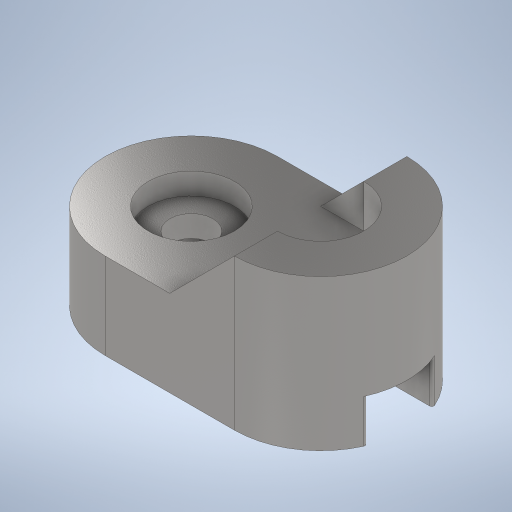
# Autodesk Inventor part: angel
Saved by Autodesk Inventor 2024 (Build 280153000, 153)
## iProperties
Created: 2024-02-01
Part Number: angel
Material: Stahl, galvanisiert
Document SubType Name: Modeling
Designer: ffogue
Density: 7.85 g/cm^3
Appearance: Galvanisiert
Author: ffogue
Autodesk Inventor part; units mm, degrees
note: some values were not read from the file. Chosen so that the rebuilt part matches the saved one: direction of "Bohrung1"; direction of "Bohrung2".
ref_plane "XY Plane" through (0, 0, 0) normal (0, 0, 1) x (1, 0, 0)
sketch "Skizze1" plane through (0, 0, 0) normal (0, 0, 1) x (1, 0, 0)
  line L0 (-70, 0) -> (70, 0) construction
  line L1 (-70, 40) -> (70, 40)
  line L2 (-70, -40) -> (70, -40)
  line L3 (-70, 40) -> (-70, -40)
  line L4 (70, 40) -> (70, -40)
  line L5 (0, 0) -> (0, 9.5703) construction
  dimension "d0" = 80
  dimension "d1" = 140
  constraints: 12 end point, 4 parallel, 2 vertical, 1 coincident, 1 horizontal, 1 midpoint, 1 vertical alignment, 2 other
  measures "d0" distance between parallel lines of L2 L1
  measures "d1" distance of L1.start L1.end
extrude "Extrusion1" add sketch "Skizze1" along normal blind 40
fillet "Rundung1" radius 40 1 edges at (-70, 40, 20)
fillet "Rundung2" radius 40 1 edges at (-70, -40, 20)
fillet "Rundung3" radius 40 1 edges at (70, 40, 20)
fillet "Rundung4" radius 40 1 edges at (70, -40, 20)
sketch "Skizze4" plane through (0, 0, 40) normal (0, 0, 1) x (1, 0, 0)
  circle A0 centre (-30, 0) radius 20
  circle A1 centre (30, 0) radius 20
  line L0 (0, 0) -> (0, 40) construction
  arc A2 (30, -40) -> (30, 40) centre (30, 0) ccw projected
  line L1 (30, 40) -> (-30, 40) projected
  point P0 (70, 0)
  dimension "d10" = 40
  dimension "d11" = 40
  dimension "d12" = 60
  constraints: 2 centre point, 2 end point, 2 horizontal alignment, 1 midpoint, 1 point on circle, 1 symmetric about line, 1 vertical
  measures "d10" diameter of A0
  measures "d11" diameter of A1
  measures "d12" distance of A1.centre A0.centre
extrude "Extrusion2" cut sketch "Skizze4" against normal blind 10
sketch "Skizze5" plane through (-30, 0, 30) normal (0, 0, 1) x (1, 0, 0)
  circle A0 centre (0, 0) radius 20 projected
  point P0 (30, 0)
  constraints: 1 coincident
hole "Bohrung1" at (-30, 0, 30) direction (0, 0, -1) diameter 20 depth 30
sketch "Skizze6" plane through (30, 0, 30) normal (0, 0, 1) x (1, 0, 0)
  circle A0 centre (0, 0) radius 20 projected
  point P0 (-30, 0)
  constraints: 1 coincident
hole "Bohrung2" at (30, 0, 30) direction (0, 0, -1) diameter 20 depth 30
sketch "Skizze7" plane through (0, 0, 40) normal (0, 0, 1) x (1, 0, 0)
  circle A0 centre (30, 0) radius 10 projected
  arc A1 (30, -40) -> (30, 40) centre (30, 0) ccw projected
  line L0 (30, 40) -> (-30, 40) projected
  arc A2 (30, -40) -> (30, 40) centre (30, 0) ccw
  circle A3 centre (30, 0) radius 20 projected
  arc A4 (30, -20) -> (30, 20) centre (30, 0) ccw
  line L1 (30, 40) -> (30, 20)
  line L2 (30, -20) -> (30, -40)
  point P0 (0, 0)
  constraints: 6 point on circle, 4 end point, 2 centre point, 2 vertical
extrude "Extrusion3" add sketch "Skizze7" along normal blind 30 contours L2 A3 L1 A1
sketch "Skizze8" plane through (-30, -40, 0) normal (0, -1, 0) x (1, 0, 0)
  line L0 (60, 40) -> (60, 70) projected
  line L1 (0, 40) -> (60, 40) projected
  line L2 (60, 70) -> (30, 40)
  line L3 (60, 40) -> (30, 40)
  line L4 (60, 40) -> (60, 70) projected
  line L5 (60, 70) -> (60, 40)
  point P0 (30, 0)
  dimension "d31" = 30
  constraints: 6 end point, 2 collinear, 1 midpoint
  measures "d31" distance of L0.start L2.end
extrude "Extrusion4" add sketch "Skizze8" against normal blind 10
ref_plane "Arbeitsebene1" through (0, 0, 0) normal (0, -1, 0) x (1, 0, 0)
mirror "Spiegeln2" about plane through (0, 0, 0) normal (0, -1, 0) of "Extrusion4"
ref_plane "Arbeitsebene3" through (0, 0, 0) normal (-1, 0, 0) x (0, -1, 0)
sketch "Skizze10" plane through (0, 0, 0) normal (-1, 0, 0) x (0, -1, 0)
  line L0 (40, 0) -> (-40, 0) projected
  line L1 (-15, 0) -> (-15, 20)
  line L2 (-15, 20) -> (15, 20)
  line L3 (15, 20) -> (15, 0)
  line L4 (0, 0) -> (0, 10) construction
  point P0 (15, 10)
  dimension "d36" = 30
  dimension "d37" = 20
  constraints: 8 end point, 2 perpendicular, 2 point on line, 2 vertical, 1 midpoint, 1 other
  measures "d36" distance from line of point (15, 10) L1
  measures "d37" distance between parallel lines of L0 L2
extrude "Extrusion5" cut sketch "Skizze10" along normal through all both and the other way through all
fillet "Rundung5" radius 1 4 edges at (-67.081, -15, 10) (-67.081, 15, 10) (67.081, 15, 10) (67.081, -15, 10)
